Autodesk Fusion 360 part; units mm, degrees
(part 38 of 40)
  spline S144 degree 5 poles (151.3635, 144.3049) (151.3327, 144.3021) (151.2711, 144.2971) (151.1787, 144.2922) (151.0554, 144.2903) (150.901, 144.2944) (150.7464, 144.3031) (150.5917, 144.3146) (150.437, 144.3277) (150.2822, 144.3417) (150.1275, 144.3569) (149.9727, 144.3735) (149.818, 144.392) (149.6632, 144.4129) (149.5085, 144.4359) (149.3538, 144.461) (149.1991, 144.4879) (149.0445, 144.5162) (148.8899, 144.5458) (148.7354, 144.5767) (148.5809, 144.6087) (148.4265, 144.6421) (148.2722, 144.6768) (148.118, 144.7129) (147.9638, 144.7503) (147.8098, 144.7891) (147.6558, 144.8291) (147.5019, 144.8703) (147.3481, 144.9127) (147.1944, 144.9561) (147.0408, 145.0007) (146.8873, 145.0464) (146.734, 145.0932) (146.5807, 145.1411) (146.4276, 145.1901) (146.2746, 145.2401) (146.1217, 145.2913) (145.9689, 145.3434) (145.8162, 145.3965) (145.6637, 145.4507) (145.5114, 145.5058) (145.3591, 145.562) (145.207, 145.619) (145.055, 145.6771) (144.9032, 145.7361) (144.7516, 145.7961) (144.6, 145.857) (144.4487, 145.9188) (144.2975, 145.9815) (144.1464, 146.0452) (143.9955, 146.1097) (143.8448, 146.1751) (143.6942, 146.2415) (143.5438, 146.3087) (143.3936, 146.3767) (143.2435, 146.4457) (143.0936, 146.5154) (142.9439, 146.5861) (142.7944, 146.6575) (142.645, 146.7299) (142.4958, 146.803) (142.3468, 146.877) (142.198, 146.9518) (142.0494, 147.0274) (141.9009, 147.1038) (141.7527, 147.181) (141.6046, 147.259) (141.4568, 147.3378) (141.3091, 147.4174) (141.1617, 147.4977) (141.0144, 147.5789) (140.8968, 147.6444) (140.8086, 147.6939) (140.7499, 147.7271) (140.7205, 147.7437) knots 0 0 0 0 0 0 0.01428571 0.02857143 0.04285714 0.05714286 0.07142857 0.08571429 0.1 0.11428571 0.12857143 0.14285714 0.15714286 0.17142857 0.18571429 0.2 0.21428571 0.22857143 0.24285714 0.25714286 0.27142857 0.28571429 0.3 0.31428571 0.32857143 0.34285714 0.35714286 0.37142857 0.38571429 0.4 0.41428571 0.42857143 0.44285714 0.45714286 0.47142857 0.48571429 0.5 0.51428571 0.52857143 0.54285714 0.55714286 0.57142857 0.58571429 0.6 0.61428571 0.62857143 0.64285714 0.65714286 0.67142857 0.68571429 0.7 0.71428571 0.72857143 0.74285714 0.75714286 0.77142857 0.78571429 0.8 0.81428571 0.82857143 0.84285714 0.85714286 0.87142857 0.88571429 0.9 0.91428571 0.92857143 0.94285714 0.95714286 0.97142857 0.98571429 1 1 1 1 1 1
  line L10797 (151.3635, 144.3049) -> (151.3327, 144.3021) construction
  line L10798 (151.3327, 144.3021) -> (151.2711, 144.2971) construction
  line L10799 (151.2711, 144.2971) -> (151.1787, 144.2922) construction
  line L10800 (151.1787, 144.2922) -> (151.0554, 144.2903) construction
  line L10801 (151.0554, 144.2903) -> (150.901, 144.2944) construction
  line L10802 (150.901, 144.2944) -> (150.7464, 144.3031) construction
  line L10803 (150.7464, 144.3031) -> (150.5917, 144.3146) construction
  line L10804 (150.5917, 144.3146) -> (150.437, 144.3277) construction
  line L10805 (150.437, 144.3277) -> (150.2822, 144.3417) construction
  line L10806 (150.2822, 144.3417) -> (150.1275, 144.3569) construction
  line L10807 (150.1275, 144.3569) -> (149.9727, 144.3735) construction
  line L10808 (149.9727, 144.3735) -> (149.818, 144.392) construction
  line L10809 (149.818, 144.392) -> (149.6632, 144.4129) construction
  line L10810 (149.6632, 144.4129) -> (149.5085, 144.4359) construction
  line L10811 (149.5085, 144.4359) -> (149.3538, 144.461) construction
  line L10812 (149.3538, 144.461) -> (149.1991, 144.4879) construction
  line L10813 (149.1991, 144.4879) -> (149.0445, 144.5162) construction
  line L10814 (149.0445, 144.5162) -> (148.8899, 144.5458) construction
  line L10815 (148.8899, 144.5458) -> (148.7354, 144.5767) construction
  line L10816 (148.7354, 144.5767) -> (148.5809, 144.6087) construction
  line L10817 (148.5809, 144.6087) -> (148.4265, 144.6421) construction
  line L10818 (148.4265, 144.6421) -> (148.2722, 144.6768) construction
  line L10819 (148.2722, 144.6768) -> (148.118, 144.7129) construction
  line L10820 (148.118, 144.7129) -> (147.9638, 144.7503) construction
  line L10821 (147.9638, 144.7503) -> (147.8098, 144.7891) construction
  line L10822 (147.8098, 144.7891) -> (147.6558, 144.8291) construction
  line L10823 (147.6558, 144.8291) -> (147.5019, 144.8703) construction
  line L10824 (147.5019, 144.8703) -> (147.3481, 144.9127) construction
  line L10825 (147.3481, 144.9127) -> (147.1944, 144.9561) construction
  line L10826 (147.1944, 144.9561) -> (147.0408, 145.0007) construction
  line L10827 (147.0408, 145.0007) -> (146.8873, 145.0464) construction
  line L10828 (146.8873, 145.0464) -> (146.734, 145.0932) construction
  line L10829 (146.734, 145.0932) -> (146.5807, 145.1411) construction
  line L10830 (146.5807, 145.1411) -> (146.4276, 145.1901) construction
  line L10831 (146.4276, 145.1901) -> (146.2746, 145.2401) construction
  line L10832 (146.2746, 145.2401) -> (146.1217, 145.2913) construction
  line L10833 (146.1217, 145.2913) -> (145.9689, 145.3434) construction
  line L10834 (145.9689, 145.3434) -> (145.8162, 145.3965) construction
  line L10835 (145.8162, 145.3965) -> (145.6637, 145.4507) construction
  line L10836 (145.6637, 145.4507) -> (145.5114, 145.5058) construction
  line L10837 (145.5114, 145.5058) -> (145.3591, 145.562) construction
  line L10838 (145.3591, 145.562) -> (145.207, 145.619) construction
  line L10839 (145.207, 145.619) -> (145.055, 145.6771) construction
  line L10840 (145.055, 145.6771) -> (144.9032, 145.7361) construction
  line L10841 (144.9032, 145.7361) -> (144.7516, 145.7961) construction
  line L10842 (144.7516, 145.7961) -> (144.6, 145.857) construction
  line L10843 (144.6, 145.857) -> (144.4487, 145.9188) construction
  line L10844 (144.4487, 145.9188) -> (144.2975, 145.9815) construction
  line L10845 (144.2975, 145.9815) -> (144.1464, 146.0452) construction
  line L10846 (144.1464, 146.0452) -> (143.9955, 146.1097) construction
  line L10847 (143.9955, 146.1097) -> (143.8448, 146.1751) construction
  line L10848 (143.8448, 146.1751) -> (143.6942, 146.2415) construction
  line L10849 (143.6942, 146.2415) -> (143.5438, 146.3087) construction
  line L10850 (143.5438, 146.3087) -> (143.3936, 146.3767) construction
  line L10851 (143.3936, 146.3767) -> (143.2435, 146.4457) construction
  line L10852 (143.2435, 146.4457) -> (143.0936, 146.5154) construction
  line L10853 (143.0936, 146.5154) -> (142.9439, 146.5861) construction
  line L10854 (142.9439, 146.5861) -> (142.7944, 146.6575) construction
  line L10855 (142.7944, 146.6575) -> (142.645, 146.7299) construction
  line L10856 (142.645, 146.7299) -> (142.4958, 146.803) construction
  line L10857 (142.4958, 146.803) -> (142.3468, 146.877) construction
  line L10858 (142.3468, 146.877) -> (142.198, 146.9518) construction
  line L10859 (142.198, 146.9518) -> (142.0494, 147.0274) construction
  line L10860 (142.0494, 147.0274) -> (141.9009, 147.1038) construction
  line L10861 (141.9009, 147.1038) -> (141.7527, 147.181) construction
  line L10862 (141.7527, 147.181) -> (141.6046, 147.259) construction
  line L10863 (141.6046, 147.259) -> (141.4568, 147.3378) construction
  line L10864 (141.4568, 147.3378) -> (141.3091, 147.4174) construction
  line L10865 (141.3091, 147.4174) -> (141.1617, 147.4977) construction
  line L10866 (141.1617, 147.4977) -> (141.0144, 147.5789) construction
  line L10867 (141.0144, 147.5789) -> (140.8968, 147.6444) construction
  line L10868 (140.8968, 147.6444) -> (140.8086, 147.6939) construction
  line L10869 (140.8086, 147.6939) -> (140.7499, 147.7271) construction
  line L10870 (140.7499, 147.7271) -> (140.7205, 147.7437) construction
  arc A284 (236.6621, 98.0646) -> (235.6801, 95.4634) centre (237.5162, 96.2562) ccw
  arc A285 (271.2762, 144.4572) -> (269.1057, 142.7194) centre (271.0895, 142.4659) ccw
  arc A286 (269.1057, 157.2806) -> (271.2762, 155.5428) centre (271.0895, 157.5341) ccw
  arc A287 (270.0943, 163.005) -> (268.567, 160.6816) centre (270.5321, 161.0535) ccw
  arc A288 (251.3803, 194.5906) -> (251.5104, 191.8132) centre (252.8816, 193.2692) ccw
  arc A289 (152.9878, 155.5428) -> (155.1583, 157.2806) centre (153.1745, 157.5341) ccw
  arc A290 (184.5338, 99.6279) -> (181.8522, 98.8934) centre (183.5728, 97.8739) ccw
  line L10871 (225.137, 207.9623) -> (225.4942, 209.5542)
  line L10872 (206.5892, 90.8558) -> (206.4369, 89.2315)
  line L10873 (217.6748, 209.1442) -> (217.8271, 210.7685)
  arc A291 (263.2386, 180.2798) -> (262.5041, 177.5982) centre (264.2581, 178.5592) ccw
  arc A292 (264.0674, 174.5301) -> (266.6686, 173.5481) centre (265.8758, 175.3842) ccw
  spline S145 degree 5 poles (152.5778, 163.3622) (152.5477, 163.369) (152.4876, 163.3833) (152.3982, 163.4071) (152.2803, 163.4435) (152.1347, 163.4951) (151.9904, 163.5511) (151.8468, 163.6099) (151.7037, 163.6701) (151.5609, 163.7313) (151.4184, 163.7935) (151.2763, 163.8571) (151.1349, 163.9226) (150.9941, 163.9902) (150.8541, 164.06) (150.7147, 164.1316) (150.5759, 164.205) (150.4376, 164.2797) (150.2998, 164.3557) (150.1623, 164.4327) (150.0253, 164.5109) (149.8888, 164.5904) (149.7528, 164.6711) (149.6172, 164.753) (149.4822, 164.8363) (149.3477, 164.9208) (149.2136, 165.0064) (149.08, 165.0932) (148.9468, 165.181) (148.814, 165.2698) (148.6817, 165.3597) (148.5499, 165.4506) (148.4185, 165.5425) (148.2875, 165.6354) (148.157, 165.7293) (148.027, 165.8242) (147.8974, 165.92) (147.7682, 166.0168) (147.6394, 166.1146) (147.5111, 166.2132) (147.3832, 166.3127) (147.2558, 166.4131) (147.1288, 166.5144) (147.0022, 166.6166) (146.876, 166.7196) (146.7503, 166.8235) (146.625, 166.9283) (146.5002, 167.0338) (146.3758, 167.1402) (146.2518, 167.2474) (146.1282, 167.3555) (146.0051, 167.4643) (145.8823, 167.5739) (145.7601, 167.6842) (145.6382, 167.7954) (145.5168, 167.9073) (145.3958, 168.02) (145.2752, 168.1335) (145.1551, 168.2477) (145.0354, 168.3626) (144.9161, 168.4782) (144.7973, 168.5946) (144.6789, 168.7118) (144.5609, 168.8296) (144.4433, 168.9481) (144.3262, 169.0674) (144.2095, 169.1873) (144.0932, 169.3079) (143.9774, 169.4293) (143.862, 169.5512) (143.747, 169.6739) (143.6553, 169.7726) (143.5868, 169.8469) (143.5412, 169.8966) (143.5184, 169.9215) knots 0 0 0 0 0 0 0.01428571 0.02857143 0.04285714 0.05714286 0.07142857 0.08571429 0.1 0.11428571 0.12857143 0.14285714 0.15714286 0.17142857 0.18571429 0.2 0.21428571 0.22857143 0.24285714 0.25714286 0.27142857 0.28571429 0.3 0.31428571 0.32857143 0.34285714 0.35714286 0.37142857 0.38571429 0.4 0.41428571 0.42857143 0.44285714 0.45714286 0.47142857 0.48571429 0.5 0.51428571 0.52857143 0.54285714 0.55714286 0.57142857 0.58571429 0.6 0.61428571 0.62857143 0.64285714 0.65714286 0.67142857 0.68571429 0.7 0.71428571 0.72857143 0.74285714 0.75714286 0.77142857 0.78571429 0.8 0.81428571 0.82857143 0.84285714 0.85714286 0.87142857 0.88571429 0.9 0.91428571 0.92857143 0.94285714 0.95714286 0.97142857 0.98571429 1 1 1 1 1 1
  line L10874 (152.5778, 163.3622) -> (152.5477, 163.369) construction
  line L10875 (152.5477, 163.369) -> (152.4876, 163.3833) construction
  line L10876 (152.4876, 163.3833) -> (152.3982, 163.4071) construction
  line L10877 (152.3982, 163.4071) -> (152.2803, 163.4435) construction
  line L10878 (152.2803, 163.4435) -> (152.1347, 163.4951) construction
  line L10879 (152.1347, 163.4951) -> (151.9904, 163.5511) construction
  line L10880 (151.9904, 163.5511) -> (151.8468, 163.6099) construction
  line L10881 (151.8468, 163.6099) -> (151.7037, 163.6701) construction
  line L10882 (151.7037, 163.6701) -> (151.5609, 163.7313) construction
  line L10883 (151.5609, 163.7313) -> (151.4184, 163.7935) construction
  line L10884 (151.4184, 163.7935) -> (151.2763, 163.8571) construction
  line L10885 (151.2763, 163.8571) -> (151.1349, 163.9226) construction
  line L10886 (151.1349, 163.9226) -> (150.9941, 163.9902) construction
  line L10887 (150.9941, 163.9902) -> (150.8541, 164.06) construction
  line L10888 (150.8541, 164.06) -> (150.7147, 164.1316) construction
  line L10889 (150.7147, 164.1316) -> (150.5759, 164.205) construction
  line L10890 (150.5759, 164.205) -> (150.4376, 164.2797) construction
  line L10891 (150.4376, 164.2797) -> (150.2998, 164.3557) construction
  line L10892 (150.2998, 164.3557) -> (150.1623, 164.4327) construction
  line L10893 (150.1623, 164.4327) -> (150.0253, 164.5109) construction
  line L10894 (150.0253, 164.5109) -> (149.8888, 164.5904) construction
  line L10895 (149.8888, 164.5904) -> (149.7528, 164.6711) construction
  line L10896 (149.7528, 164.6711) -> (149.6172, 164.753) construction
  line L10897 (149.6172, 164.753) -> (149.4822, 164.8363) construction
  line L10898 (149.4822, 164.8363) -> (149.3477, 164.9208) construction
  line L10899 (149.3477, 164.9208) -> (149.2136, 165.0064) construction
  line L10900 (149.2136, 165.0064) -> (149.08, 165.0932) construction
  line L10901 (149.08, 165.0932) -> (148.9468, 165.181) construction
  line L10902 (148.9468, 165.181) -> (148.814, 165.2698) construction
  line L10903 (148.814, 165.2698) -> (148.6817, 165.3597) construction
  line L10904 (148.6817, 165.3597) -> (148.5499, 165.4506) construction
  line L10905 (148.5499, 165.4506) -> (148.4185, 165.5425) construction
  line L10906 (148.4185, 165.5425) -> (148.2875, 165.6354) construction
  line L10907 (148.2875, 165.6354) -> (148.157, 165.7293) construction
  line L10908 (148.157, 165.7293) -> (148.027, 165.8242) construction
  line L10909 (148.027, 165.8242) -> (147.8974, 165.92) construction
  line L10910 (147.8974, 165.92) -> (147.7682, 166.0168) construction
  line L10911 (147.7682, 166.0168) -> (147.6394, 166.1146) construction
  line L10912 (147.6394, 166.1146) -> (147.5111, 166.2132) construction
  line L10913 (147.5111, 166.2132) -> (147.3832, 166.3127) construction
  line L10914 (147.3832, 166.3127) -> (147.2558, 166.4131) construction
  line L10915 (147.2558, 166.4131) -> (147.1288, 166.5144) construction
  line L10916 (147.1288, 166.5144) -> (147.0022, 166.6166) construction
  line L10917 (147.0022, 166.6166) -> (146.876, 166.7196) construction
  line L10918 (146.876, 166.7196) -> (146.7503, 166.8235) construction
  line L10919 (146.7503, 166.8235) -> (146.625, 166.9283) construction
  line L10920 (146.625, 166.9283) -> (146.5002, 167.0338) construction
  line L10921 (146.5002, 167.0338) -> (146.3758, 167.1402) construction
  line L10922 (146.3758, 167.1402) -> (146.2518, 167.2474) construction
  line L10923 (146.2518, 167.2474) -> (146.1282, 167.3555) construction
  line L10924 (146.1282, 167.3555) -> (146.0051, 167.4643) construction
  line L10925 (146.0051, 167.4643) -> (145.8823, 167.5739) construction
  line L10926 (145.8823, 167.5739) -> (145.7601, 167.6842) construction
  line L10927 (145.7601, 167.6842) -> (145.6382, 167.7954) construction
  line L10928 (145.6382, 167.7954) -> (145.5168, 167.9073) construction
  line L10929 (145.5168, 167.9073) -> (145.3958, 168.02) construction
  line L10930 (145.3958, 168.02) -> (145.2752, 168.1335) construction
  line L10931 (145.2752, 168.1335) -> (145.1551, 168.2477) construction
  line L10932 (145.1551, 168.2477) -> (145.0354, 168.3626) construction
  line L10933 (145.0354, 168.3626) -> (144.9161, 168.4782) construction
  line L10934 (144.9161, 168.4782) -> (144.7973, 168.5946) construction
  line L10935 (144.7973, 168.5946) -> (144.6789, 168.7118) construction
  line L10936 (144.6789, 168.7118) -> (144.5609, 168.8296) construction
  line L10937 (144.5609, 168.8296) -> (144.4433, 168.9481) construction
  line L10938 (144.4433, 168.9481) -> (144.3262, 169.0674) construction
  line L10939 (144.3262, 169.0674) -> (144.2095, 169.1873) construction
  line L10940 (144.2095, 169.1873) -> (144.0932, 169.3079) construction
  line L10941 (144.0932, 169.3079) -> (143.9774, 169.4293) construction
  line L10942 (143.9774, 169.4293) -> (143.862, 169.5512) construction
  line L10943 (143.862, 169.5512) -> (143.747, 169.6739) construction
  line L10944 (143.747, 169.6739) -> (143.6553, 169.7726) construction
  line L10945 (143.6553, 169.7726) -> (143.5868, 169.8469) construction
  line L10946 (143.5868, 169.8469) -> (143.5412, 169.8966) construction
  line L10947 (143.5412, 169.8966) -> (143.5184, 169.9215) construction
  spline S146 degree 5 poles (156.0975, 174.1948) (156.0692, 174.2071) (156.0122, 174.2308) (155.9258, 174.264) (155.8091, 174.3039) (155.6609, 174.3478) (155.5112, 174.3873) (155.3606, 174.4241) (155.2094, 174.4595) (155.0579, 174.494) (154.906, 174.5274) (154.7537, 174.5594) (154.6008, 174.5896) (154.4472, 174.6176) (154.2929, 174.6435) (154.138, 174.6674) (153.9826, 174.6897) (153.8268, 174.7105) (153.6706, 174.7301) (153.5141, 174.7485) (153.3573, 174.7658) (153.2002, 174.7818) (153.0427, 174.7965) (152.8849, 174.8098) (152.7267, 174.8218) (152.5682, 174.8325) (152.4094, 174.842) (152.2503, 174.8504) (152.0909, 174.8577) (151.9313, 174.8638) (151.7715, 174.8689) (151.6114, 174.8729) (151.4511, 174.8757) (151.2905, 174.8776) (151.1297, 174.8783) (150.9687, 174.878) (150.8075, 174.8766) (150.6461, 174.8742) (150.4845, 174.8708) (150.3227, 174.8665) (150.1608, 174.8611) (149.9986, 174.8548) (149.8363, 174.8475) (149.6739, 174.8392) (149.5113, 174.83) (149.3485, 174.8199) (149.1856, 174.8088) (149.0225, 174.7967) (148.8593, 174.7838) (148.696, 174.77) (148.5325, 174.7552) (148.3689, 174.7396) (148.2052, 174.723) (148.0414, 174.7056) (147.8775, 174.6873) (147.7135, 174.6681) (147.5494, 174.648) (147.3852, 174.6271) (147.2209, 174.6054) (147.0565, 174.5828) (146.892, 174.5593) (146.7274, 174.535) (146.5628, 174.5098) (146.398, 174.4839) (146.2333, 174.4571) (146.0684, 174.4294) (145.9035, 174.401) (145.7385, 174.3718) (145.5735, 174.3417) (145.4084, 174.3108) (145.2433, 174.2792) (145.1112, 174.2532) (145.0121, 174.2334) (144.946, 174.22) (144.9129, 174.2132) knots 0 0 0 0 0 0 0.01428571 0.02857143 0.04285714 0.05714286 0.07142857 0.08571429 0.1 0.11428571 0.12857143 0.14285714 0.15714286 0.17142857 0.18571429 0.2 0.21428571 0.22857143 0.24285714 0.25714286 0.27142857 0.28571429 0.3 0.31428571 0.32857143 0.34285714 0.35714286 0.37142857 0.38571429 0.4 0.41428571 0.42857143 0.44285714 0.45714286 0.47142857 0.48571429 0.5 0.51428571 0.52857143 0.54285714 0.55714286 0.57142857 0.58571429 0.6 0.61428571 0.62857143 0.64285714 0.65714286 0.67142857 0.68571429 0.7 0.71428571 0.72857143 0.74285714 0.75714286 0.77142857 0.78571429 0.8 0.81428571 0.82857143 0.84285714 0.85714286 0.87142857 0.88571429 0.9 0.91428571 0.92857143 0.94285714 0.95714286 0.97142857 0.98571429 1 1 1 1 1 1
  line L10948 (156.0975, 174.1948) -> (156.0692, 174.2071) construction
  line L10949 (156.0692, 174.2071) -> (156.0122, 174.2308) construction
  line L10950 (156.0122, 174.2308) -> (155.9258, 174.264) construction
  line L10951 (155.9258, 174.264) -> (155.8091, 174.3039) construction
  line L10952 (155.8091, 174.3039) -> (155.6609, 174.3478) construction
  line L10953 (155.6609, 174.3478) -> (155.5112, 174.3873) construction
  line L10954 (155.5112, 174.3873) -> (155.3606, 174.4241) construction
  line L10955 (155.3606, 174.4241) -> (155.2094, 174.4595) construction
  line L10956 (155.2094, 174.4595) -> (155.0579, 174.494) construction
  line L10957 (155.0579, 174.494) -> (154.906, 174.5274) construction
  line L10958 (154.906, 174.5274) -> (154.7537, 174.5594) construction
  line L10959 (154.7537, 174.5594) -> (154.6008, 174.5896) construction
  line L10960 (154.6008, 174.5896) -> (154.4472, 174.6176) construction
  line L10961 (154.4472, 174.6176) -> (154.2929, 174.6435) construction
  line L10962 (154.2929, 174.6435) -> (154.138, 174.6674) construction
  line L10963 (154.138, 174.6674) -> (153.9826, 174.6897) construction
  line L10964 (153.9826, 174.6897) -> (153.8268, 174.7105) construction
  line L10965 (153.8268, 174.7105) -> (153.6706, 174.7301) construction
  line L10966 (153.6706, 174.7301) -> (153.5141, 174.7485) construction
  line L10967 (153.5141, 174.7485) -> (153.3573, 174.7658) construction
  line L10968 (153.3573, 174.7658) -> (153.2002, 174.7818) construction
  line L10969 (153.2002, 174.7818) -> (153.0427, 174.7965) construction
  line L10970 (153.0427, 174.7965) -> (152.8849, 174.8098) construction
  line L10971 (152.8849, 174.8098) -> (152.7267, 174.8218) construction
  line L10972 (152.7267, 174.8218) -> (152.5682, 174.8325) construction
  line L10973 (152.5682, 174.8325) -> (152.4094, 174.842) construction
  line L10974 (152.4094, 174.842) -> (152.2503, 174.8504) construction
  line L10975 (152.2503, 174.8504) -> (152.0909, 174.8577) construction
  line L10976 (152.0909, 174.8577) -> (151.9313, 174.8638) construction
  line L10977 (151.9313, 174.8638) -> (151.7715, 174.8689) construction
  line L10978 (151.7715, 174.8689) -> (151.6114, 174.8729) construction
  line L10979 (151.6114, 174.8729) -> (151.4511, 174.8757) construction
  line L10980 (151.4511, 174.8757) -> (151.2905, 174.8776) construction
  line L10981 (151.2905, 174.8776) -> (151.1297, 174.8783) construction
  line L10982 (151.1297, 174.8783) -> (150.9687, 174.878) construction
  line L10983 (150.9687, 174.878) -> (150.8075, 174.8766) construction
  line L10984 (150.8075, 174.8766) -> (150.6461, 174.8742) construction
  line L10985 (150.6461, 174.8742) -> (150.4845, 174.8708) construction
  line L10986 (150.4845, 174.8708) -> (150.3227, 174.8665) construction
  line L10987 (150.3227, 174.8665) -> (150.1608, 174.8611) construction
  line L10988 (150.1608, 174.8611) -> (149.9986, 174.8548) construction
  line L10989 (149.9986, 174.8548) -> (149.8363, 174.8475) construction
  line L10990 (149.8363, 174.8475) -> (149.6739, 174.8392) construction
  line L10991 (149.6739, 174.8392) -> (149.5113, 174.83) construction
  line L10992 (149.5113, 174.83) -> (149.3485, 174.8199) construction
  line L10993 (149.3485, 174.8199) -> (149.1856, 174.8088) construction
  line L10994 (149.1856, 174.8088) -> (149.0225, 174.7967) construction
  line L10995 (149.0225, 174.7967) -> (148.8593, 174.7838) construction
  line L10996 (148.8593, 174.7838) -> (148.696, 174.77) construction
  line L10997 (148.696, 174.77) -> (148.5325, 174.7552) construction
  line L10998 (148.5325, 174.7552) -> (148.3689, 174.7396) construction
  line L10999 (148.3689, 174.7396) -> (148.2052, 174.723) construction
  line L11000 (148.2052, 174.723) -> (148.0414, 174.7056) construction
  line L11001 (148.0414, 174.7056) -> (147.8775, 174.6873) construction
  line L11002 (147.8775, 174.6873) -> (147.7135, 174.6681) construction
  line L11003 (147.7135, 174.6681) -> (147.5494, 174.648) construction
  line L11004 (147.5494, 174.648) -> (147.3852, 174.6271) construction
  line L11005 (147.3852, 174.6271) -> (147.2209, 174.6054) construction
  line L11006 (147.2209, 174.6054) -> (147.0565, 174.5828) construction
  line L11007 (147.0565, 174.5828) -> (146.892, 174.5593) construction
  line L11008 (146.892, 174.5593) -> (146.7274, 174.535) construction
  line L11009 (146.7274, 174.535) -> (146.5628, 174.5098) construction
  line L11010 (146.5628, 174.5098) -> (146.398, 174.4839) construction
  line L11011 (146.398, 174.4839) -> (146.2333, 174.4571) construction
  line L11012 (146.2333, 174.4571) -> (146.0684, 174.4294) construction
  line L11013 (146.0684, 174.4294) -> (145.9035, 174.401) construction
  line L11014 (145.9035, 174.401) -> (145.7385, 174.3718) construction
  line L11015 (145.7385, 174.3718) -> (145.5735, 174.3417) construction
  line L11016 (145.5735, 174.3417) -> (145.4084, 174.3108) construction
  line L11017 (145.4084, 174.3108) -> (145.2433, 174.2792) construction
  line L11018 (145.2433, 174.2792) -> (145.1112, 174.2532) construction
  line L11019 (145.1112, 174.2532) -> (145.0121, 174.2334) construction
  line L11020 (145.0121, 174.2334) -> (144.946, 174.22) construction
  line L11021 (144.946, 174.22) -> (144.9129, 174.2132) construction
  arc A293 (222.8136, 206.435) -> (219.4126, 206.9737) centre (212.132, 150) ccw
  spline S147 degree 5 poles (271.6862, 163.3622) (271.7163, 163.369) (271.7764, 163.3833) (271.8658, 163.4071) (271.9837, 163.4435) (272.1293, 163.4951) (272.2736, 163.5511) (272.4172, 163.6099) (272.5603, 163.6701) (272.7031, 163.7313) (272.8456, 163.7935) (272.9877, 163.8571) (273.1291, 163.9226) (273.2699, 163.9902) (273.4099, 164.06) (273.5493, 164.1316) (273.6881, 164.205) (273.8264, 164.2797) (273.9642, 164.3557) (274.1017, 164.4327) (274.2387, 164.5109) (274.3752, 164.5904) (274.5112, 164.6711) (274.6468, 164.753) (274.7818, 164.8363) (274.9163, 164.9208) (275.0504, 165.0064) (275.184, 165.0932) (275.3172, 165.181) (275.45, 165.2698) (275.5823, 165.3597) (275.7141, 165.4506) (275.8455, 165.5425) (275.9765, 165.6354) (276.107, 165.7293) (276.237, 165.8242) (276.3666, 165.92) (276.4958, 166.0168) (276.6246, 166.1146) (276.7529, 166.2132) (276.8808, 166.3127) (277.0082, 166.4131) (277.1352, 166.5144) (277.2618, 166.6166) (277.388, 166.7196) (277.5137, 166.8235) (277.639, 166.9283) (277.7638, 167.0338) (277.8882, 167.1402) (278.0122, 167.2474) (278.1358, 167.3555) (278.2589, 167.4643) (278.3817, 167.5739) (278.5039, 167.6842) (278.6258, 167.7954) (278.7472, 167.9073) (278.8682, 168.02) (278.9888, 168.1335) (279.1089, 168.2477) (279.2286, 168.3626) (279.3479, 168.4782) (279.4667, 168.5946) (279.5851, 168.7118) (279.7031, 168.8296) (279.8207, 168.9481) (279.9378, 169.0674) (280.0545, 169.1873) (280.1708, 169.3079) (280.2866, 169.4293) (280.402, 169.5512) (280.517, 169.6739) (280.6087, 169.7726) (280.6772, 169.8469) (280.7228, 169.8966) (280.7456, 169.9215) knots 0 0 0 0 0 0 0.01428571 0.02857143 0.04285714 0.05714286 0.07142857 0.08571429 0.1 0.11428571 0.12857143 0.14285714 0.15714286 0.17142857 0.18571429 0.2 0.21428571 0.22857143 0.24285714 0.25714286 0.27142857 0.28571429 0.3 0.31428571 0.32857143 0.34285714 0.35714286 0.37142857 0.38571429 0.4 0.41428571 0.42857143 0.44285714 0.45714286 0.47142857 0.48571429 0.5 0.51428571 0.52857143 0.54285714 0.55714286 0.57142857 0.58571429 0.6 0.61428571 0.62857143 0.64285714 0.65714286 0.67142857 0.68571429 0.7 0.71428571 0.72857143 0.74285714 0.75714286 0.77142857 0.78571429 0.8 0.81428571 0.82857143 0.84285714 0.85714286 0.87142857 0.88571429 0.9 0.91428571 0.92857143 0.94285714 0.95714286 0.97142857 0.98571429 1 1 1 1 1 1
  line L11022 (271.6862, 163.3622) -> (271.7163, 163.369) construction
  line L11023 (271.7163, 163.369) -> (271.7764, 163.3833) construction
  line L11024 (271.7764, 163.3833) -> (271.8658, 163.4071) construction
  line L11025 (271.8658, 163.4071) -> (271.9837, 163.4435) construction
  line L11026 (271.9837, 163.4435) -> (272.1293, 163.4951) construction
  line L11027 (272.1293, 163.4951) -> (272.2736, 163.5511) construction
  line L11028 (272.2736, 163.5511) -> (272.4172, 163.6099) construction
  line L11029 (272.4172, 163.6099) -> (272.5603, 163.6701) construction
  line L11030 (272.5603, 163.6701) -> (272.7031, 163.7313) construction
  line L11031 (272.7031, 163.7313) -> (272.8456, 163.7935) construction
  line L11032 (272.8456, 163.7935) -> (272.9877, 163.8571) construction
  line L11033 (272.9877, 163.8571) -> (273.1291, 163.9226) construction
  line L11034 (273.1291, 163.9226) -> (273.2699, 163.9902) construction
  line L11035 (273.2699, 163.9902) -> (273.4099, 164.06) construction
  line L11036 (273.4099, 164.06) -> (273.5493, 164.1316) construction
  line L11037 (273.5493, 164.1316) -> (273.6881, 164.205) construction
  line L11038 (273.6881, 164.205) -> (273.8264, 164.2797) construction
  line L11039 (273.8264, 164.2797) -> (273.9642, 164.3557) construction
  line L11040 (273.9642, 164.3557) -> (274.1017, 164.4327) construction
  line L11041 (274.1017, 164.4327) -> (274.2387, 164.5109) construction
  line L11042 (274.2387, 164.5109) -> (274.3752, 164.5904) construction
  line L11043 (274.3752, 164.5904) -> (274.5112, 164.6711) construction
  line L11044 (274.5112, 164.6711) -> (274.6468, 164.753) construction
  line L11045 (274.6468, 164.753) -> (274.7818, 164.8363) construction
  line L11046 (274.7818, 164.8363) -> (274.9163, 164.9208) construction
  line L11047 (274.9163, 164.9208) -> (275.0504, 165.0064) construction
  line L11048 (275.0504, 165.0064) -> (275.184, 165.0932) construction
  line L11049 (275.184, 165.0932) -> (275.3172, 165.181) construction
  line L11050 (275.3172, 165.181) -> (275.45, 165.2698) construction
  line L11051 (275.45, 165.2698) -> (275.5823, 165.3597) construction
  line L11052 (275.5823, 165.3597) -> (275.7141, 165.4506) construction
  line L11053 (275.7141, 165.4506) -> (275.8455, 165.5425) construction
  line L11054 (275.8455, 165.5425) -> (275.9765, 165.6354) construction
  line L11055 (275.9765, 165.6354) -> (276.107, 165.7293) construction
  line L11056 (276.107, 165.7293) -> (276.237, 165.8242) construction
  line L11057 (276.237, 165.8242) -> (276.3666, 165.92) construction
  line L11058 (276.3666, 165.92) -> (276.4958, 166.0168) construction
  line L11059 (276.4958, 166.0168) -> (276.6246, 166.1146) construction
  line L11060 (276.6246, 166.1146) -> (276.7529, 166.2132) construction
  line L11061 (276.7529, 166.2132) -> (276.8808, 166.3127) construction
  line L11062 (276.8808, 166.3127) -> (277.0082, 166.4131) construction
  line L11063 (277.0082, 166.4131) -> (277.1352, 166.5144) construction
  line L11064 (277.1352, 166.5144) -> (277.2618, 166.6166) construction
  line L11065 (277.2618, 166.6166) -> (277.388, 166.7196) construction
  line L11066 (277.388, 166.7196) -> (277.5137, 166.8235) construction
  line L11067 (277.5137, 166.8235) -> (277.639, 166.9283) construction
  line L11068 (277.639, 166.9283) -> (277.7638, 167.0338) construction
  line L11069 (277.7638, 167.0338) -> (277.8882, 167.1402) construction
  line L11070 (277.8882, 167.1402) -> (278.0122, 167.2474) construction
  line L11071 (278.0122, 167.2474) -> (278.1358, 167.3555) construction
  line L11072 (278.1358, 167.3555) -> (278.2589, 167.4643) construction
  line L11073 (278.2589, 167.4643) -> (278.3817, 167.5739) construction
  line L11074 (278.3817, 167.5739) -> (278.5039, 167.6842) construction
  line L11075 (278.5039, 167.6842) -> (278.6258, 167.7954) construction
  line L11076 (278.6258, 167.7954) -> (278.7472, 167.9073) construction
  line L11077 (278.7472, 167.9073) -> (278.8682, 168.02) construction
  line L11078 (278.8682, 168.02) -> (278.9888, 168.1335) construction
  line L11079 (278.9888, 168.1335) -> (279.1089, 168.2477) construction
  line L11080 (279.1089, 168.2477) -> (279.2286, 168.3626) construction
  line L11081 (279.2286, 168.3626) -> (279.3479, 168.4782) construction
  line L11082 (279.3479, 168.4782) -> (279.4667, 168.5946) construction
  line L11083 (279.4667, 168.5946) -> (279.5851, 168.7118) construction
  line L11084 (279.5851, 168.7118) -> (279.7031, 168.8296) construction
  line L11085 (279.7031, 168.8296) -> (279.8207, 168.9481) construction
  line L11086 (279.8207, 168.9481) -> (279.9378, 169.0674) construction
  line L11087 (279.9378, 169.0674) -> (280.0545, 169.1873) construction
  line L11088 (280.0545, 169.1873) -> (280.1708, 169.3079) construction
  line L11089 (280.1708, 169.3079) -> (280.2866, 169.4293) construction
  line L11090 (280.2866, 169.4293) -> (280.402, 169.5512) construction
  line L11091 (280.402, 169.5512) -> (280.517, 169.6739) construction
  line L11092 (280.517, 169.6739) -> (280.6087, 169.7726) construction
  line L11093 (280.6087, 169.7726) -> (280.6772, 169.8469) construction
  line L11094 (280.6772, 169.8469) -> (280.7228, 169.8966) construction
  line L11095 (280.7228, 169.8966) -> (280.7456, 169.9215) construction
  circle A294 centre (212.132, 150) radius 2.3
  arc A295 (239.7302, 200.3721) -> (236.6621, 201.9354) centre (212.132, 150) ccw
  arc A296 (269.1057, 157.2806) -> (268.567, 160.6816) centre (212.132, 150) ccw
  arc A297 (201.4504, 93.565) -> (204.8514, 93.0263) centre (212.132, 150) ccw
  spline S148 degree 5 poles (198.7698, 90.4458) (198.763, 90.4157) (198.7487, 90.3556) (198.7249, 90.2662) (198.6885, 90.1483) (198.6369, 90.0027) (198.5809, 89.8584) (198.5221, 89.7148) (198.4619, 89.5717) (198.4007, 89.4289) (198.3385, 89.2864) (198.2749, 89.1443) (198.2094, 89.0029) (198.1418, 88.8621) (198.072, 88.7221) (198.0004, 88.5827) (197.927, 88.4439) (197.8523, 88.3056) (197.7763, 88.1678) (197.6993, 88.0303) (197.6211, 87.8933) (197.5416, 87.7568) (197.4609, 87.6208) (197.379, 87.4852) (197.2957, 87.3502) (197.2112, 87.2157) (197.1256, 87.0816) (197.0388, 86.948) (196.951, 86.8148) (196.8622, 86.682) (196.7723, 86.5497) (196.6814, 86.4179) (196.5895, 86.2865) (196.4966, 86.1555) (196.4027, 86.025) (196.3078, 85.895) (196.212, 85.7654) (196.1152, 85.6362) (196.0174, 85.5074) (195.9188, 85.3791) (195.8193, 85.2512) (195.7189, 85.1238) (195.6176, 84.9968) (195.5154, 84.8702) (195.4124, 84.744) (195.3085, 84.6183) (195.2037, 84.493) (195.0982, 84.3682) (194.9918, 84.2438) (194.8846, 84.1198) (194.7765, 83.9962) (194.6677, 83.8731) (194.5581, 83.7503) (194.4478, 83.6281) (194.3366, 83.5062) (194.2247, 83.3848) (194.112, 83.2638) (193.9985, 83.1432) (193.8843, 83.0231) (193.7694, 82.9034) (193.6538, 82.7841) (193.5374, 82.6653) (193.4202, 82.5469) (193.3024, 82.4289) (193.1839, 82.3113) (193.0646, 82.1942) (192.9447, 82.0775) (192.8241, 81.9612) (192.7027, 81.8454) (192.5808, 81.73) (192.4581, 81.615) (192.3594, 81.5233) (192.2851, 81.4548) (192.2354, 81.4092) (192.2105, 81.3864) knots 0 0 0 0 0 0 0.01428571 0.02857143 0.04285714 0.05714286 0.07142857 0.08571429 0.1 0.11428571 0.12857143 0.14285714 0.15714286 0.17142857 0.18571429 0.2 0.21428571 0.22857143 0.24285714 0.25714286 0.27142857 0.28571429 0.3 0.31428571 0.32857143 0.34285714 0.35714286 0.37142857 0.38571429 0.4 0.41428571 0.42857143 0.44285714 0.45714286 0.47142857 0.48571429 0.5 0.51428571 0.52857143 0.54285714 0.55714286 0.57142857 0.58571429 0.6 0.61428571 0.62857143 0.64285714 0.65714286 0.67142857 0.68571429 0.7 0.71428571 0.72857143 0.74285714 0.75714286 0.77142857 0.78571429 0.8 0.81428571 0.82857143 0.84285714 0.85714286 0.87142857 0.88571429 0.9 0.91428571 0.92857143 0.94285714 0.95714286 0.97142857 0.98571429 1 1 1 1 1 1
  line L11096 (198.7698, 90.4458) -> (198.763, 90.4157) construction
  line L11097 (198.763, 90.4157) -> (198.7487, 90.3556) construction
  line L11098 (198.7487, 90.3556) -> (198.7249, 90.2662) construction
  line L11099 (198.7249, 90.2662) -> (198.6885, 90.1483) construction
  line L11100 (198.6885, 90.1483) -> (198.6369, 90.0027) construction
  line L11101 (198.6369, 90.0027) -> (198.5809, 89.8584) construction
  line L11102 (198.5809, 89.8584) -> (198.5221, 89.7148) construction
  line L11103 (198.5221, 89.7148) -> (198.4619, 89.5717) construction
  line L11104 (198.4619, 89.5717) -> (198.4007, 89.4289) construction
  line L11105 (198.4007, 89.4289) -> (198.3385, 89.2864) construction
  line L11106 (198.3385, 89.2864) -> (198.2749, 89.1443) construction
  line L11107 (198.2749, 89.1443) -> (198.2094, 89.0029) construction
  line L11108 (198.2094, 89.0029) -> (198.1418, 88.8621) construction
  line L11109 (198.1418, 88.8621) -> (198.072, 88.7221) construction
  line L11110 (198.072, 88.7221) -> (198.0004, 88.5827) construction
  line L11111 (198.0004, 88.5827) -> (197.927, 88.4439) construction
  line L11112 (197.927, 88.4439) -> (197.8523, 88.3056) construction
  line L11113 (197.8523, 88.3056) -> (197.7763, 88.1678) construction
  line L11114 (197.7763, 88.1678) -> (197.6993, 88.0303) construction
  line L11115 (197.6993, 88.0303) -> (197.6211, 87.8933) construction
  line L11116 (197.6211, 87.8933) -> (197.5416, 87.7568) construction
  line L11117 (197.5416, 87.7568) -> (197.4609, 87.6208) construction
  line L11118 (197.4609, 87.6208) -> (197.379, 87.4852) construction
  line L11119 (197.379, 87.4852) -> (197.2957, 87.3502) construction
  line L11120 (197.2957, 87.3502) -> (197.2112, 87.2157) construction
  line L11121 (197.2112, 87.2157) -> (197.1256, 87.0816) construction
  line L11122 (197.1256, 87.0816) -> (197.0388, 86.948) construction
  line L11123 (197.0388, 86.948) -> (196.951, 86.8148) construction
  line L11124 (196.951, 86.8148) -> (196.8622, 86.682) construction
  line L11125 (196.8622, 86.682) -> (196.7723, 86.5497) construction
  line L11126 (196.7723, 86.5497) -> (196.6814, 86.4179) construction
  line L11127 (196.6814, 86.4179) -> (196.5895, 86.2865) construction
  line L11128 (196.5895, 86.2865) -> (196.4966, 86.1555) construction
  line L11129 (196.4966, 86.1555) -> (196.4027, 86.025) construction
  line L11130 (196.4027, 86.025) -> (196.3078, 85.895) construction
  line L11131 (196.3078, 85.895) -> (196.212, 85.7654) construction
  line L11132 (196.212, 85.7654) -> (196.1152, 85.6362) construction
  line L11133 (196.1152, 85.6362) -> (196.0174, 85.5074) construction
  line L11134 (196.0174, 85.5074) -> (195.9188, 85.3791) construction
  line L11135 (195.9188, 85.3791) -> (195.8193, 85.2512) construction
  line L11136 (195.8193, 85.2512) -> (195.7189, 85.1238) construction
  line L11137 (195.7189, 85.1238) -> (195.6176, 84.9968) construction
  line L11138 (195.6176, 84.9968) -> (195.5154, 84.8702) construction
  line L11139 (195.5154, 84.8702) -> (195.4124, 84.744) construction
  line L11140 (195.4124, 84.744) -> (195.3085, 84.6183) construction
  line L11141 (195.3085, 84.6183) -> (195.2037, 84.493) construction
  line L11142 (195.2037, 84.493) -> (195.0982, 84.3682) construction
  line L11143 (195.0982, 84.3682) -> (194.9918, 84.2438) construction
  line L11144 (194.9918, 84.2438) -> (194.8846, 84.1198) construction
  line L11145 (194.8846, 84.1198) -> (194.7765, 83.9962) construction
  line L11146 (194.7765, 83.9962) -> (194.6677, 83.8731) construction
  line L11147 (194.6677, 83.8731) -> (194.5581, 83.7503) construction
  line L11148 (194.5581, 83.7503) -> (194.4478, 83.6281) construction
  line L11149 (194.4478, 83.6281) -> (194.3366, 83.5062) construction
  line L11150 (194.3366, 83.5062) -> (194.2247, 83.3848) construction
  line L11151 (194.2247, 83.3848) -> (194.112, 83.2638) construction
  line L11152 (194.112, 83.2638) -> (193.9985, 83.1432) construction
  line L11153 (193.9985, 83.1432) -> (193.8843, 83.0231) construction
  line L11154 (193.8843, 83.0231) -> (193.7694, 82.9034) construction
  line L11155 (193.7694, 82.9034) -> (193.6538, 82.7841) construction
  line L11156 (193.6538, 82.7841) -> (193.5374, 82.6653) construction
  line L11157 (193.5374, 82.6653) -> (193.4202, 82.5469) construction
  line L11158 (193.4202, 82.5469) -> (193.3024, 82.4289) construction
  line L11159 (193.3024, 82.4289) -> (193.1839, 82.3113) construction
  line L11160 (193.1839, 82.3113) -> (193.0646, 82.1942) construction
  line L11161 (193.0646, 82.1942) -> (192.9447, 82.0775) construction
  line L11162 (192.9447, 82.0775) -> (192.8241, 81.9612) construction
  line L11163 (192.8241, 81.9612) -> (192.7027, 81.8454) construction
  line L11164 (192.7027, 81.8454) -> (192.5808, 81.73) construction
  line L11165 (192.5808, 81.73) -> (192.4581, 81.615) construction
  line L11166 (192.4581, 81.615) -> (192.3594, 81.5233) construction
  line L11167 (192.3594, 81.5233) -> (192.2851, 81.4548) construction
  line L11168 (192.2851, 81.4548) -> (192.2354, 81.4092) construction
  line L11169 (192.2354, 81.4092) -> (192.2105, 81.3864) construction
  arc A298 (222.8136, 206.435) -> (225.137, 207.9623) centre (223.1855, 208.4001) ccw
  arc A299 (172.8837, 105.4094) -> (172.7536, 108.1868) centre (171.3824, 106.7308) ccw
  arc A300 (184.5338, 99.6279) -> (187.6019, 98.0646) centre (212.132, 150) ccw
  spline S149 degree 5 poles (171.8057, 195.8153) (171.7853, 195.8385) (171.7452, 195.8854) (171.6869, 195.9573) (171.6128, 196.056) (171.5254, 196.1833) (171.4416, 196.3135) (171.36, 196.4454) (171.2796, 196.5782) (171.2, 196.7117) (171.1213, 196.8458) (171.0437, 196.9807) (170.9678, 197.1168) (170.8937, 197.2543) (170.8214, 197.393) (170.7507, 197.5329) (170.6816, 197.6738) (170.6136, 197.8156) (170.5467, 197.9581) (170.4808, 198.1012) (170.416, 198.245) (170.3522, 198.3895) (170.2896, 198.5347) (170.2281, 198.6807) (170.1678, 198.8274) (170.1086, 198.9749) (170.0505, 199.123) (169.9934, 199.2717) (169.9373, 199.421) (169.8821, 199.5709) (169.8279, 199.7214) (169.7746, 199.8724) (169.7223, 200.024) (169.671, 200.1761) (169.6206, 200.3288) (169.5712, 200.482) (169.5226, 200.6358) (169.475, 200.79) (169.4283, 200.9447) (169.3825, 201.0999) (169.3375, 201.2556) (169.2934, 201.4118) (169.2502, 201.5684) (169.2079, 201.7255) (169.1664, 201.883) (169.1257, 202.0409) (169.0859, 202.1993) (169.047, 202.3581) (169.0089, 202.5173) (168.9716, 202.6769) (168.9351, 202.8369) (168.8994, 202.9973) (168.8646, 203.1581) (168.8305, 203.3193) (168.7973, 203.4809) (168.7648, 203.6428) (168.7332, 203.8051) (168.7023, 203.9677) (168.6723, 204.1307) (168.643, 204.294) (168.6145, 204.4577) (168.5867, 204.6217) (168.5597, 204.7861) (168.5336, 204.9508) (168.5081, 205.1158) (168.4834, 205.2811) (168.4595, 205.4467) (168.4364, 205.6126) (168.414, 205.7789) (168.3923, 205.9454) (168.3714, 206.1122) (168.3553, 206.2459) (168.3435, 206.3463) (168.3358, 206.4133) (168.332, 206.4469) knots 0 0 0 0 0 0 0.01428571 0.02857143 0.04285714 0.05714286 0.07142857 0.08571429 0.1 0.11428571 0.12857143 0.14285714 0.15714286 0.17142857 0.18571429 0.2 0.21428571 0.22857143 0.24285714 0.25714286 0.27142857 0.28571429 0.3 0.31428571 0.32857143 0.34285714 0.35714286 0.37142857 0.38571429 0.4 0.41428571 0.42857143 0.44285714 0.45714286 0.47142857 0.48571429 0.5 0.51428571 0.52857143 0.54285714 0.55714286 0.57142857 0.58571429 0.6 0.61428571 0.62857143 0.64285714 0.65714286 0.67142857 0.68571429 0.7 0.71428571 0.72857143 0.74285714 0.75714286 0.77142857 0.78571429 0.8 0.81428571 0.82857143 0.84285714 0.85714286 0.87142857 0.88571429 0.9 0.91428571 0.92857143 0.94285714 0.95714286 0.97142857 0.98571429 1 1 1 1 1 1
  line L11170 (171.8057, 195.8153) -> (171.7853, 195.8385) construction
  line L11171 (171.7853, 195.8385) -> (171.7452, 195.8854) construction
  line L11172 (171.7452, 195.8854) -> (171.6869, 195.9573) construction
  line L11173 (171.6869, 195.9573) -> (171.6128, 196.056) construction
  line L11174 (171.6128, 196.056) -> (171.5254, 196.1833) construction
  line L11175 (171.5254, 196.1833) -> (171.4416, 196.3135) construction
  line L11176 (171.4416, 196.3135) -> (171.36, 196.4454) construction
  line L11177 (171.36, 196.4454) -> (171.2796, 196.5782) construction
  line L11178 (171.2796, 196.5782) -> (171.2, 196.7117) construction
  line L11179 (171.2, 196.7117) -> (171.1213, 196.8458) construction
  line L11180 (171.1213, 196.8458) -> (171.0437, 196.9807) construction
  line L11181 (171.0437, 196.9807) -> (170.9678, 197.1168) construction
  line L11182 (170.9678, 197.1168) -> (170.8937, 197.2543) construction
  line L11183 (170.8937, 197.2543) -> (170.8214, 197.393) construction
  line L11184 (170.8214, 197.393) -> (170.7507, 197.5329) construction
  line L11185 (170.7507, 197.5329) -> (170.6816, 197.6738) construction
  line L11186 (170.6816, 197.6738) -> (170.6136, 197.8156) construction
  line L11187 (170.6136, 197.8156) -> (170.5467, 197.9581) construction
  line L11188 (170.5467, 197.9581) -> (170.4808, 198.1012) construction
  line L11189 (170.4808, 198.1012) -> (170.416, 198.245) construction
  line L11190 (170.416, 198.245) -> (170.3522, 198.3895) construction
  line L11191 (170.3522, 198.3895) -> (170.2896, 198.5347) construction
  line L11192 (170.2896, 198.5347) -> (170.2281, 198.6807) construction
  line L11193 (170.2281, 198.6807) -> (170.1678, 198.8274) construction
  line L11194 (170.1678, 198.8274) -> (170.1086, 198.9749) construction
  line L11195 (170.1086, 198.9749) -> (170.0505, 199.123) construction
  line L11196 (170.0505, 199.123) -> (169.9934, 199.2717) construction
  line L11197 (169.9934, 199.2717) -> (169.9373, 199.421) construction
  line L11198 (169.9373, 199.421) -> (169.8821, 199.5709) construction
  line L11199 (169.8821, 199.5709) -> (169.8279, 199.7214) construction
  line L11200 (169.8279, 199.7214) -> (169.7746, 199.8724) construction
  line L11201 (169.7746, 199.8724) -> (169.7223, 200.024) construction
  line L11202 (169.7223, 200.024) -> (169.671, 200.1761) construction
  line L11203 (169.671, 200.1761) -> (169.6206, 200.3288) construction
  line L11204 (169.6206, 200.3288) -> (169.5712, 200.482) construction
  line L11205 (169.5712, 200.482) -> (169.5226, 200.6358) construction
  line L11206 (169.5226, 200.6358) -> (169.475, 200.79) construction
  line L11207 (169.475, 200.79) -> (169.4283, 200.9447) construction
  line L11208 (169.4283, 200.9447) -> (169.3825, 201.0999) construction
  line L11209 (169.3825, 201.0999) -> (169.3375, 201.2556) construction
  line L11210 (169.3375, 201.2556) -> (169.2934, 201.4118) construction
  line L11211 (169.2934, 201.4118) -> (169.2502, 201.5684) construction
  line L11212 (169.2502, 201.5684) -> (169.2079, 201.7255) construction
  line L11213 (169.2079, 201.7255) -> (169.1664, 201.883) construction
  line L11214 (169.1664, 201.883) -> (169.1257, 202.0409) construction
  line L11215 (169.1257, 202.0409) -> (169.0859, 202.1993) construction
  line L11216 (169.0859, 202.1993) -> (169.047, 202.3581) construction
  line L11217 (169.047, 202.3581) -> (169.0089, 202.5173) construction
  line L11218 (169.0089, 202.5173) -> (168.9716, 202.6769) construction
  line L11219 (168.9716, 202.6769) -> (168.9351, 202.8369) construction
  line L11220 (168.9351, 202.8369) -> (168.8994, 202.9973) construction
  line L11221 (168.8994, 202.9973) -> (168.8646, 203.1581) construction
  line L11222 (168.8646, 203.1581) -> (168.8305, 203.3193) construction
  line L11223 (168.8305, 203.3193) -> (168.7973, 203.4809) construction
  line L11224 (168.7973, 203.4809) -> (168.7648, 203.6428) construction
  line L11225 (168.7648, 203.6428) -> (168.7332, 203.8051) construction
  line L11226 (168.7332, 203.8051) -> (168.7023, 203.9677) construction
  line L11227 (168.7023, 203.9677) -> (168.6723, 204.1307) construction
  line L11228 (168.6723, 204.1307) -> (168.643, 204.294) construction
  line L11229 (168.643, 204.294) -> (168.6145, 204.4577) construction
  line L11230 (168.6145, 204.4577) -> (168.5867, 204.6217) construction
  line L11231 (168.5867, 204.6217) -> (168.5597, 204.7861) construction
  line L11232 (168.5597, 204.7861) -> (168.5336, 204.9508) construction
  line L11233 (168.5336, 204.9508) -> (168.5081, 205.1158) construction
  line L11234 (168.5081, 205.1158) -> (168.4834, 205.2811) construction
  line L11235 (168.4834, 205.2811) -> (168.4595, 205.4467) construction
  line L11236 (168.4595, 205.4467) -> (168.4364, 205.6126) construction
  line L11237 (168.4364, 205.6126) -> (168.414, 205.7789) construction
  line L11238 (168.414, 205.7789) -> (168.3923, 205.9454) construction
  line L11239 (168.3923, 205.9454) -> (168.3714, 206.1122) construction
  line L11240 (168.3714, 206.1122) -> (168.3553, 206.2459) construction
  line L11241 (168.3553, 206.2459) -> (168.3435, 206.3463) construction
  line L11242 (168.3435, 206.3463) -> (168.3358, 206.4133) construction
  line L11243 (168.3358, 206.4133) -> (168.332, 206.4469) construction
  arc A301 (242.4118, 98.8934) -> (239.7302, 99.6279) centre (240.6912, 97.8739) ccw
  spline S150 degree 5 poles (159.6217, 181.1115) (159.5952, 181.1272) (159.5425, 181.1594) (159.4648, 181.2097) (159.3639, 181.2807) (159.2414, 181.3748) (159.1214, 181.4727) (159.0031, 181.5729) (158.8856, 181.6744) (158.7686, 181.7767) (158.6523, 181.88) (158.5369, 181.9844) (158.4226, 182.0903) (158.3096, 182.1981) (158.198, 182.3077) (158.0876, 182.419) (157.9783, 182.5316) (157.8698, 182.6455) (157.7622, 182.7603) (157.6553, 182.876) (157.5492, 182.9927) (157.4439, 183.1105) (157.3394, 183.2292) (157.2359, 183.3491) (157.1332, 183.47) (157.0313, 183.5919) (156.9303, 183.7148) (156.83, 183.8386) (156.7305, 183.9633) (156.6317, 184.0888) (156.5336, 184.2151) (156.4363, 184.3423) (156.3397, 184.4703) (156.2439, 184.5991) (156.1488, 184.7288) (156.0544, 184.8592) (155.9608, 184.9905) (155.8678, 185.1224) (155.7756, 185.2552) (155.684, 185.3886) (155.5932, 185.5228) (155.503, 185.6577) (155.4135, 185.7933) (155.3247, 185.9295) (155.2365, 186.0665) (155.1491, 186.2042) (155.0623, 186.3425) (154.9762, 186.4815) (154.8907, 186.6211) (154.8059, 186.7614) (154.7218, 186.9023) (154.6383, 187.0438) (154.5555, 187.186) (154.4733, 187.3288) (154.3917, 187.4721) (154.3108, 187.6161) (154.2306, 187.7607) (154.151, 187.9058) (154.072, 188.0515) (153.9937, 188.1978) (153.916, 188.3447) (153.8389, 188.4921) (153.7625, 188.6401) (153.6867, 188.7886) (153.6115, 188.9377) (153.537, 189.0873) (153.463, 189.2374) (153.3897, 189.3881) (153.3171, 189.5393) (153.245, 189.6909) (153.1736, 189.8431) (153.1169, 189.9653) (153.0747, 190.0572) (153.0467, 190.1185) (153.0327, 190.1492) knots 0 0 0 0 0 0 0.01428571 0.02857143 0.04285714 0.05714286 0.07142857 0.08571429 0.1 0.11428571 0.12857143 0.14285714 0.15714286 0.17142857 0.18571429 0.2 0.21428571 0.22857143 0.24285714 0.25714286 0.27142857 0.28571429 0.3 0.31428571 0.32857143 0.34285714 0.35714286 0.37142857 0.38571429 0.4 0.41428571 0.42857143 0.44285714 0.45714286 0.47142857 0.48571429 0.5 0.51428571 0.52857143 0.54285714 0.55714286 0.57142857 0.58571429 0.6 0.61428571 0.62857143 0.64285714 0.65714286 0.67142857 0.68571429 0.7 0.71428571 0.72857143 0.74285714 0.75714286 0.77142857 0.78571429 0.8 0.81428571 0.82857143 0.84285714 0.85714286 0.87142857 0.88571429 0.9 0.91428571 0.92857143 0.94285714 0.95714286 0.97142857 0.98571429 1 1 1 1 1 1
  line L11244 (159.6217, 181.1115) -> (159.5952, 181.1272) construction
  line L11245 (159.5952, 181.1272) -> (159.5425, 181.1594) construction
  line L11246 (159.5425, 181.1594) -> (159.4648, 181.2097) construction
  line L11247 (159.4648, 181.2097) -> (159.3639, 181.2807) construction
  line L11248 (159.3639, 181.2807) -> (159.2414, 181.3748) construction
  line L11249 (159.2414, 181.3748) -> (159.1214, 181.4727) construction
  line L11250 (159.1214, 181.4727) -> (159.0031, 181.5729) construction